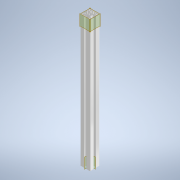
# Autodesk Inventor part: 10-540
Saved by Autodesk Inventor 2022 (Build 260153000, 153)
## iProperties
Created: 2004-09-16
Part Number: 10-540
Material: Alluminio - 6061
Document SubType Name: Modeling
Designer: Chapin
Manufacturer: Standard
Standards Organization: Custom
Mass: 299.838 g
Surface Area: 1133.85 cm^2
Volume: 110.641 cm^3
Density: 2.71 g/cm^3
Appearance: Alluminio - Piatto
LastFilename: Not Set
Author: Chapin
Autodesk Inventor part; units mm, degrees
ref_plane "YZ Plane" through (0, 0, 0) normal (1, 0, 0) x (0, 1, 0)
ref_plane "XZ Plane" through (0, 0, 0) normal (0, 1, 0) x (-1, 0, 0)
ref_plane "XY Plane" through (0, 0, 0) normal (0, 0, 1) x (1, 0, 0)
sketch "Sketch1" plane through (0, 0, 0) normal (0, 0, 1) x (1, 0, 0)
  line L0 (-20, 20) -> (20, 20)
  line L1 (20, 20) -> (20, -20)
  line L2 (20, -20) -> (-20, -20)
  line L3 (-20, -20) -> (-20, 20)
  point P0 (0, 0)
  dimension "d0" = 40
  dimension "d1" = 40
  dimension "d2" = 20
  dimension "d3" = 20
  constraints: 8 end point, 2 parallel, 1 horizontal, 1 perpendicular
  measures "d0" distance of L0.start L0.end
  measures "d1" distance of L2.end L0.start
  measures "d2" distance from line of point (0, 0) L3
  measures "d3" distance from line of point (0, 0) L0
extrude "Extrusion1" add sketch "Sketch1" against normal blind 540
sketch "Sketch2" plane through (0, 0, 0) normal (0, 0, 1) x (1, 0, 0)
  line L0 (-20, 20) -> (20, 20) projected
  line L1 (0, -28.1243) -> (0, 28.7456) projected
  line L2 (-20, 17) -> (-20, -20)
  line L3 (-17, 20) -> (20, 20)
  arc A0 (-17, 20) -> (-20, 17) centre (-17, 17) ccw
  line L4 (-17, 20) -> (-4.065, 19.5483)
  line L5 (-4.065, 19.5483) -> (-4.065, 15.5)
  line L6 (-4.065, 15.5) -> (-6.645, 15.5)
  line L7 (-6.645, 15.5) -> (-6.645, 18)
  line L8 (-6.645, 18) -> (-10.65, 18)
  line L9 (-10.65, 18) -> (-10.65, 13.832)
  line L10 (-10.65, 13.832) -> (-4.068, 7.25)
  line L11 (-4.068, 7.25) -> (0, 7.25)
  line L12 (17, 20) -> (4.065, 19.5483)
  line L13 (4.065, 19.5483) -> (4.065, 15.5)
  line L14 (4.065, 15.5) -> (6.645, 15.5)
  line L15 (6.645, 15.5) -> (6.645, 18)
  line L16 (6.645, 18) -> (10.65, 18)
  line L17 (10.65, 18) -> (10.65, 13.832)
  line L18 (10.65, 13.832) -> (4.068, 7.25)
  line L19 (4.068, 7.25) -> (0, 7.25)
  line L20 (-17, 20) -> (17, 20)
  line L21 (-20, 20) -> (0, 0)
  dimension "d6" = 3
  dimension "d10" = 2
  dimension "d11" = 8.13
  dimension "d12" = 21.3
  dimension "d13" = 7.25
  dimension "d15" = 4.5
  dimension "d16" = 2
  dimension "d21" = 2.25
  dimension "d24" = 2.58
  constraints: 40 end point, 8 symmetric about line, 5 perpendicular, 3 parallel, 3 point on line, 3 tangent, 2 collinear, 2 point on circle, 1 centre point
  measures "d6" radius of A0
  measures "d10" angle of L0 L4
  measures "d11" diameter of L5 L1
  measures "d12" diameter of L9 L1
  measures "d13" distance from line of L21.end L11
  measures "d15" distance between parallel lines of L0 L6
  measures "d16" distance between parallel lines of L3 L8
  measures "d21" distance between parallel lines of L21 L10
  measures "d24" distance between parallel lines of L5 L7
extrude "Extrusion2" cut sketch "Sketch2" against normal through all contours L0 L1 L11 L10 L9 L8 L7 L6 L5 L4 | L0 L12 L13 L14 L15 L16 L17 L18 L19 L1
fillet "Fillet1" radius 1 4 edges at (-4.065, 19.5483, -270) (4.065, 19.5483, -270) (-4.068, 7.25, -270) (4.068, 7.25, -270)
fillet "Fillet2" radius 2 4 edges at (-6.645, 18, -270) (-10.65, 18, -270) (6.645, 18, -270) (10.65, 18, -270)
fillet "Fillet3" radius 4 2 edges at (-10.65, 13.832, -270) (10.65, 13.832, -270)
fillet "Fillet4" radius 0.5 4 edges at (-6.645, 15.5, -270) (-4.065, 15.5, -270) (4.065, 15.5, -270) (6.645, 15.5, -270)
pattern_circular "Circular Pattern1" count 4 over 360 about axis through (0, 0, -10) along (0, 0, 1) of "Extrusion2", "Fillet1", "Fillet2", "Fillet3", "Fillet4"
fillet "Fillet5" radius 3 4 edges at (-20, 20, -270) (20, 20, -270) (20, -20, -270) (-20, -20, -270)
sketch "Sketch3" plane through (0, 0, 0) normal (0, 0, 1) x (1, 0, 0)
  point P0 (0, 0)
hole "Hole1" at (0, 0, 0) direction (0, 0, -1) diameter 6.7 end through all
sketch "Sketch4" plane through (0, 0, 0) normal (0, 0, 1) x (1, 0, 0)
  circle A0 centre (0, 0) radius 3.35 projected
  line L0 (-4.3609, 7.5429) -> (-9.4784, 12.6604) projected
  arc A1 (-10.65, 15.4888) -> (-9.4784, 12.6604) centre (-6.65, 15.4888) ccw projected
  line L1 (-10.65, 15.4888) -> (-10.65, 16) projected
  arc A2 (-8.65, 18) -> (-10.65, 16) centre (-8.65, 16) ccw projected
  line L2 (-5.0301, 19.582) -> (-17, 20) projected
  arc A3 (-17, 20) -> (-20, 17) centre (-17, 17) ccw projected
  line L3 (-20, 17) -> (-19.582, 5.0301) projected
  arc A4 (-16, 10.65) -> (-18, 8.65) centre (-16, 8.65) ccw projected
  line L4 (-16, 10.65) -> (-15.4888, 10.65) projected
  arc A5 (-12.6604, 9.4784) -> (-15.4888, 10.65) centre (-15.4888, 6.65) ccw projected
  line L5 (-18.4798, 17.0219) -> (-18.2811, 11.3309)
  arc A6 (-17, 18.48) -> (-18.4798, 17.0219) centre (-17, 17) ccw
  line L6 (-11.3309, 18.2811) -> (-17.0219, 18.4798)
  arc A7 (-11.3309, 18.2811) -> (-12.17, 16) centre (-8.65, 16) ccw
  arc A8 (-12.17, 15.4888) -> (-11.0395, 12.1418) centre (-6.65, 15.4888) ccw
  arc A9 (-16, 12.17) -> (-18.2811, 11.3309) centre (-16, 8.65) ccw
  arc A10 (-12.1418, 11.0395) -> (-15.4888, 12.17) centre (-15.4888, 6.65) ccw
  line L7 (-16, 12.17) -> (-15.4888, 12.17)
  line L8 (-12.17, 15.4888) -> (-12.17, 16)
  line L9 (-12.1418, 11.0395) -> (-11.0395, 12.1418)
  line L10 (-17, 17) -> (0, 0)
  line L11 (-17, 17) -> (-19.1213, 19.1213)
  dimension "d38" = 1.52
  dimension "d39" = 1.52
  dimension "d40" = 1.52
  dimension "d41" = 1.52
  dimension "d42" = 1.52
  dimension "d43" = 1.52
  dimension "d44" = 1.52
  dimension "d45" = 1.52
  dimension "d46" = 1.52
  dimension "d47" = 10.65
  constraints: 14 end point, 12 point on circle, 5 centre point, 4 parallel, 2 perpendicular, 1 collinear
  measures "d38" distance between parallel lines of L2 L6
  measures "d39" radial gap between concentric circles of A3 A6
  measures "d40" distance between parallel lines of L3 L5
  measures "d41" radial gap between concentric circles of A4 A9
  measures "d42" distance between parallel lines of L4 L7
  measures "d43" radial gap between concentric circles of A5 A10
  measures "d44" radial gap between concentric circles of A1 A8
  measures "d45" distance between parallel lines of L1 L8
  measures "d46" radial gap between concentric circles of A2 A7
  measures "d47" distance from line of L9 L11.end
extrude "Extrusion3" cut sketch "Sketch4" against normal through all contours L9 A10 L7 A9 L5 A6 L11 L10 | L10 L11 A6 L6 A7 L8 A8 L9
fillet "Fillet6" radius 1 2 edges at (-18.2811, 11.3309, -270) (-11.3309, 18.2811, -270)
fillet "Fillet6" radius 0.38 2 edges at (-11.0395, 12.1418, -270) (-12.1418, 11.0395, -270)
pattern_circular "Circular Pattern2" count 4 over 360 about axis through (0, 0, -10) along (0, 0, 1) of "Extrusion3", "Fillet6"
sketch "Sketch5" plane through (0, 0, 0) normal (0, 0, 1) x (1, 0, 0)
  circle A0 centre (0, 0) radius 3.35 projected
  arc A1 (-17, 20) -> (-20, 17) centre (-17, 17) ccw projected
  line L0 (4.3609, -7.5429) -> (9.4784, -12.6604) projected
  line L1 (0, 0) -> (-17, 17)
  arc A2 (-2.0186, 5.6502) -> (-5.6502, 2.0186) centre (0, 0) ccw
  line L2 (-11.1937, 9.838) -> (-5.6502, 4.2946)
  line L3 (-11.5906, 11.5906) -> (-10.9128, 12.2685)
  line L4 (-11.1937, 9.838) -> (-9.838, 11.1937)
  line L5 (-4.2946, 5.6502) -> (-2.0186, 5.6502)
  line L6 (-5.6502, 4.2946) -> (-5.6502, 2.0186)
  line L7 (-9.838, 11.1937) -> (-4.2946, 5.6502)
  line L8 (-11.2677, 11.9136) -> (-11.9136, 11.2677) projected
  dimension "d54" = 12
  dimension "d55" = 1.52
  dimension "d56" = 90
  dimension "d57" = 45
  dimension "d59" = 2.276
  dimension "d60" = 1.9172
  dimension "d67" = 0.9586
  constraints: 14 end point, 4 parallel, 2 perpendicular, 2 point on circle, 1 centre point, 1 coincident, 1 collinear, 1 point on line
  measures "d54" diameter of A2
  measures "d55" distance between parallel lines of L4 L3
  measures "d56" angle of L5 L6
  measures "d57" angle of L5 L1
  measures "d59" distance of L5.start L5.end
  measures "d60" distance between parallel lines of L2 L7
  measures "d67" distance between parallel lines of L1 L7
extrude "Extrusion4" cut sketch "Sketch5" against normal through all contours A2 L6 L2 L4 L1 | L1 L4 L7 L5 A2
fillet "Fillet7" radius 0.38 4 edges at (-2.0186, 5.6502, -270) (-5.6502, 2.0186, -270) (-9.838, 11.1937, -270) (-11.1937, 9.838, -270)
pattern_circular "Circular Pattern3" count 4 over 360 about axis through (0, 0, -10) along (0, 0, 1) of "Extrusion4", "Fillet7"
ref_plane "T-Slot1" through (0, 18.5826, -540) normal (1, 0, 0) x (0, 1, 0)
ref_plane "T-Slot2" through (16, 0, -540) normal (0, 1, 0) x (-1, 0, 0)
ref_plane "Side1" through (-20, 17, 0) normal (-1, 0, 0) x (0, -1, 0)
ref_plane "Side2" through (17, 20, 0) normal (0, 1, 0) x (-1, 0, 0)
ref_plane "Side3" through (20, -17, 0) normal (1, 0, 0) x (0, 1, 0)
ref_plane "Side4" through (-17, -20, 0) normal (0, -1, 0) x (1, 0, 0)
equation "\"d2\" = 0.5 * d0"
equation "\"d3\" = 0.5 * d1"
equation "\"d67\" = 0.5 * d60"
